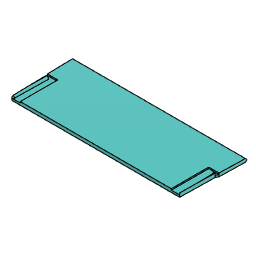
Drawer Divider Akro-Mils Organizer A2 (Autodesk Fusion 360 design; units mm, degrees)
Autodesk Fusion 360 part; units mm, degrees
sketch "Sketch1" plane through (0, 0, 0) normal (0, 0, 1) x (1, 0, 0)
  line L0 (-65, -25) -> (65, -25)
  line L1 (65, -25) -> (65.5, 2)
  line L2 (65.5, 2) -> (66.5, 4)
  line L3 (66.5, 4) -> (67, 25)
  line L4 (67, 25) -> (-67, 25)
  line L5 (-67, 25) -> (-66.5, 4)
  line L6 (-66.5, 4) -> (-65.5, 2)
  line L7 (-65.5, 2) -> (-65, -25)
  line L8 (0, 25) -> (0, -25) construction
  line L9 (-65.5, 2) -> (65.5, 2) construction
  line L10 (66.5, 4) -> (-66.5, 4)
  line L11 (-65.5, 2) -> (-63.5, 2)
  line L12 (-63.5, 2) -> (-64, -25)
  line L13 (65.5, 2) -> (63.5, 2)
  line L14 (63.5, 2) -> (64, -25)
  line L15 (-58.5, 25) -> (-58.5, -25)
  line L16 (58.5, 25) -> (58.5, -25)
  point P0 (0, 2)
  point P1 (0, 4)
  dimension "d1" = 130
  dimension "d2" = 131
  dimension "d3" = 27
  dimension "d4" = 29
  dimension "d5" = 50
  dimension "d6" = 134
  dimension "d7" = 133
  dimension "d8" = 1
  dimension "d9" = 2
  dimension "d10" = 1
  dimension "d11" = 2
  dimension "d22" = 8
  dimension "d23" = 8
  constraint horizontal L0
  constraint midpoint L4 L8.start
  constraint midpoint L0 L8.end
  constraint horizontal L4
  constraint vertical L8
  constraint midpoint L8 origin
  constraint horizontal L9
  constraint horizontal L10
  constraint midpoint L9 P0
  constraint midpoint L10 P1
  constraint coincident L8 P1
  constraint coincident L8 P0
  constraint coincident L9 L11.end
  constraint parallel L9 L11
  constraint coincident L0 L12.end
  constraint coincident L9 L13.end
  constraint parallel L9 L13
  constraint coincident L0 L14.end
  constraint coincident L4 L15.start
  constraint coincident L0 L15.end
  constraint perpendicular L0 L15
  constraint coincident L4 L16.start
  constraint coincident L0 L16.end
  constraint perpendicular L0 L16
  measures "d1" distance of L0.start L0.end
  measures "d2" distance of L1.end L6.end
  measures "d3" distance of L0 L9
  measures "d4" distance of L0 L10
  measures "d5" distance of L0 L4
  measures "d6" distance of L3.end L4.end
  measures "d7" distance of L2.end L5.end
  measures "d8" distance of L0.start L12.end
  measures "d9" distance of L6.end L11.end
  measures "d10" distance of L0.end L14.end
  measures "d11" distance of L1.end L13.end
  measures "d22" distance of L5.end L15
  measures "d23" distance of L2.end L16
extrude "Extrude1" add sketch "Sketch1" along normal blind 1.5 contours L0 L7 L11 L12 | L0 L1 L13 L14 makes body 1 at (-65.3333, -7, 0.5) makes body 2 at (63.6667, -7, 0.5)
extrude "Extrude3" add sketch "Sketch1" along normal blind 1 separate body contours L0 L10 L15 L16 | L4 L5 L10 L15 | L4 L10 L15 L16 | L3 L4 L10 L16 makes body 3
extrude "Extrude2" add sketch "Sketch1" against normal blind 1.5 bodies 1 3 2
fillet "Fillet1" radius 1.5 2 edges at (-63.75, -11.5, 1.5) (63.75, -11.5, 1.5) on bodies 1
chamfer "Chamfer1" distance 1 angle 45 2 edges at (0, 25, -1.5) (0, 25, 1) on bodies 1
fillet "Fillet2" radius 1 2 edges at (-64.2752, -25, 0.866) (64.2752, -25, 0.866) on bodies 1
equation "d10 = d8"
equation "d11 = d9"
equation "d23 = d22"
